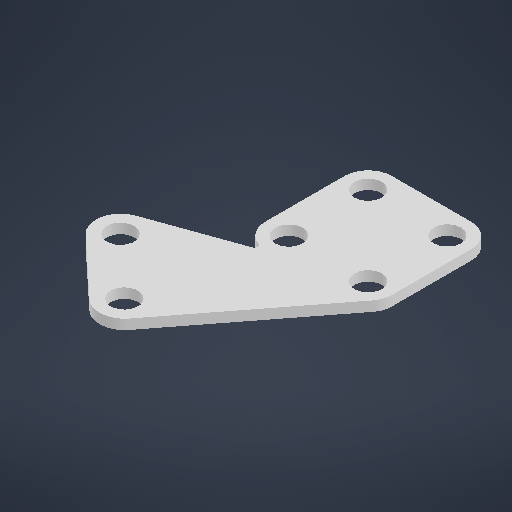
# Autodesk Inventor part: lbMountInside
Saved by Autodesk Inventor 2025.2 (Build 292293000, 293)
## iProperties
Created: 2025-03-24
Part Number: lbMountInside
Material: Generic
Document SubType Name: Modeling
Designer: Jahan
Density: 1 g/cm^3
Appearance: Default
Author: Jahan
Autodesk Inventor part; units mm, degrees
ref_plane "YZ Plane" through (0, 0, 0) normal (1, 0, 0) x (0, 1, 0)
ref_plane "XZ Plane" through (0, 0, 0) normal (0, 1, 0) x (-1, 0, 0)
ref_plane "XY Plane" through (0, 0, 0) normal (0, 0, 1) x (1, 0, 0)
sketch "Sketch1" plane through (0, 0, 0) normal (0, 1, 0) x (-1, 0, 0)
  ellipse E0 centre (13.1478, 12.5921) end of major axis (11.6568, 10.9957) minor radius 2.1844
  ellipse E1 centre (3.8663, 21.2606) end of major axis (2.3753, 19.6642) minor radius 2.1844
  circle A0 centre (-0.5698, -0.6484) radius 2.1844
  circle A1 centre (-0.5733, -13.3589) radius 2.1844
  circle A2 centre (-13.2733, -13.3589) radius 2.1844
  circle A3 centre (-13.2733, -0.6589) radius 2.1844
  line L0 (-17.0833, -0.6589) -> (-17.0833, -13.3598)
  line L1 (-13.2733, -17.1689) -> (-0.5733, -17.1689)
  line L2 (3.2367, -13.3589) -> (3.2367, -0.6589)
  arc A4 (3.2367, -0.6589) -> (0.6585, 2.9465) centre (-0.5733, -0.6589) ccw
  arc A5 (-0.5733, -17.1689) -> (3.2367, -13.3589) centre (-0.5733, -13.3589) ccw
  arc A6 (-16.4762, 1.4045) -> (-17.0833, -0.6589) centre (-13.2733, -0.6589) ccw
  arc A7 (-17.0833, -13.3598) -> (-13.2733, -17.1689) centre (-13.2733, -13.3589) ccw
  line L3 (6.5646, 24.1645) -> (15.84, 15.5017)
  line L4 (0.7159, 23.679) -> (-16.4762, 1.4045)
  line L5 (0.6551, 3.9093) -> (14.4839, 8.8603)
  arc A8 (0.6551, 3.9093) -> (0.6585, 2.9465) centre (0.8272, 3.4285) ccw
  arc A9 (14.4839, 8.8603) -> (15.84, 15.5017) centre (13.1268, 12.5966) ccw
  arc A10 (6.5646, 24.1645) -> (0.7159, 23.679) centre (3.862, 21.2507) ccw
  point P0 (0, 0)
  constraints: 14 point on circle, 12 end point, 11 centre point, 4 coincident, 3 tangent, 1 vertical, 6 other
extrude "Extrusion1" add sketch "Sketch1" along normal blind 1.5875
body "Solid1"
